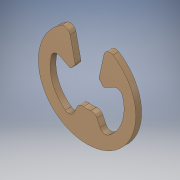
# Autodesk Inventor part: E-Clip
Saved by Autodesk Inventor 2019 (Build 230136000, 136)
## iProperties
Created: 2019-11-20
Part Number: E-Clip
Material: Generic
Document SubType Name: Modeling
Designer: Jopa
Density: 1 g/cm^3
Appearance: Brindle
Author: Jopa
Autodesk Inventor part; units mm, degrees
ref_plane "YZ Plane" through (0, 0, 0) normal (1, 0, 0) x (0, 1, 0)
ref_plane "XZ Plane" through (0, 0, 0) normal (0, 1, 0) x (-1, 0, 0)
ref_plane "XY Plane" through (0, 0, 0) normal (0, 0, 1) x (1, 0, 0)
sketch "Sketch1" plane through (0, 0, 0) normal (0, 0, 1) x (1, 0, 0)
  circle A0 centre (0, 0) radius 1.1906
  circle A1 centre (0, 0) radius 3.175
  dimension "d0" = 2.3813
  dimension "d1" = 6.35
  constraints: 2 centre point, 2 coincident
  measures "d0" diameter of A0
  measures "d1" diameter of A1
extrude "Extrusion1" add sketch "Sketch1" along normal mid plane 0.381
sketch "Sketch2" plane through (0, 0, 0.1905) normal (0, 0, 1) x (1, 0, 0)
  circle A0 centre (0, 0) radius 1.1906 construction
  circle A1 centre (0, 0) radius 3.175 projected
  line L0 (0, -4.445) -> (0, 4.445) projected
  line L1 (-4.445, 0) -> (4.445, 0) projected
  circle A2 centre (0, 0) radius 1.1906 construction
  line L2 (-0.635, 0.3107) -> (0.635, 0.3107)
  line L3 (0.635, 0.3107) -> (1.27, 3.175)
  line L4 (1.27, 3.175) -> (-1.27, 3.175)
  line L5 (-1.27, 3.175) -> (-0.635, 0.3107)
  circle A3 centre (0, 0) radius 3.175 projected
  dimension "d4" = 1.27
  dimension "d5" = 2.54
  dimension "d6" = 25
  constraints: 8 end point, 1 horizontal, 1 parallel, 1 tangent, 1 other
  measures "d4" distance of L2.start L2.end
  measures "d5" distance of L3.end L4.end
  measures "d6" angle of L3 L5
extrude "Extrusion2" cut sketch "Sketch2" against normal through all contours L3 L2 L0 A1 | A1 L4 L3 | L0 L2 L5 A1 | A1 L5 L4
sketch "Sketch3" plane through (0, 0, 0.1905) normal (0, 0, 1) x (1, 0, 0)
  arc A0 (-1.2163, 2.9328) -> (1.2163, 2.9328) centre (0, 0) ccw projected
  arc A1 (-2.1409, 1.1132) -> (2.1409, 1.1132) centre (0, 0) ccw
  line L0 (-4.445, 0) -> (4.445, 0) projected
  line L1 (0, -4.3966) -> (0, 4.1543) projected
  line L2 (-2.1409, 1.1132) -> (-1.0566, 0.5487)
  arc A2 (-0.7678, 0.9099) -> (0.7678, 0.9099) centre (0, 0) ccw projected
  line L3 (2.1409, 1.1132) -> (1.0566, 0.5487)
  line L4 (-0.7678, 0.9099) -> (-1.2163, 2.9328) projected
  line L5 (-0.5029, -1.0792) -> (-1.0195, -2.187)
  line L6 (0.5029, -1.0792) -> (1.0195, -2.187)
  dimension "d9" = 0.762
  dimension "d10" = 50
  dimension "d11" = 50
  dimension "d12" = 2.1133
  dimension "d13" = 1.0058
  constraints: 8 end point, 8 point on circle, 1 centre point, 2 other
  measures "d9" radial gap between concentric circles of A0 A1
  measures "d10" angle of L4 L2
  measures "d11" angle of L6 L5
  measures "d12" distance of L3.end L2.end
  measures "d13" distance of L6.start L5.start
extrude "Extrusion3" cut sketch "Sketch3" against normal through all contours L0 A2 L5 A1 | A1 L2 A2 L0 | L0 A2 L3 A1 | A1 L6 A2 L0
fillet "Fillet1" radius 0.381 8 edges at (-1.2163, 2.9328, 0) (1.2163, 2.9328, 0) (-2.1409, 1.1132, 0) (2.1409, 1.1132, 0) (-1.0195, -2.187, 0) (1.0195, -2.187, 0) (0.5029, -1.0792, 0) (-0.5029, -1.0792, 0)
fillet "Fillet2" radius 0.127 4 edges at (-0.7678, 0.9099, 0) (-1.0566, 0.5487, 0) (0.7678, 0.9099, 0) (1.0566, 0.5487, 0)
body "Solid1"
